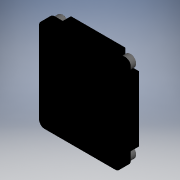
# Autodesk Inventor part: SCHUNK-Deckel ERD
Saved by Autodesk Inventor 2017.3 (Build 213256000, 256)
## iProperties
Part Number: SCHUNK-Deckel ERD
Material: Generic
Catalog Web Link: www.cadenas.de
Description: Deckel-Miniature rotary unit
Vendor: SCHUNK
Document SubType Name: Modeling
Designer: partserver
Manufacturer: SCHUNK
Mass: 53.3739 g
Surface Area: 125.943 cm^2
Volume: 53.3739 cm^3
Density: 1 g/cm^3
Appearance: PSOLRGB-0-0-0
Category: PARTsolutions
Company: SCHUNK
Title: SCHUNK-ERD
Author: Cadenas PARTsolutions
Comments: Miniature rotary unit
PSOL_IDENT_0: {$CADENAS_DATA\23d-libs\schunk\greifsysteme\drehmodule\drehmodule_elektrisch\schwenkeinheiten\miniat
PSOL_IDENT_1: ur_schwenkeinheiten\erd_dec.prj},167 {VTYP=3D},{NB=SCHUNK-Deckel ERD},{LINA=SCHUNK-ERD},{NN=Deckel},
PSOL_IDENT_2: {DATE=23.04.2020 15:23:31},{GEOMDATE=04.12.2019 08:06:04},{VERSION=},{LINEID=10},{WBVAR=},{WBNUMERIC=
PSOL_IDENT_3: }  {NB=SCHUNK-Deckel ERD},{LINA=SCHUNK-ERD},{KT=DUMMY},{TYP=ERD},{L=68.000},{B=60.000},{H1=15.000},{
PSOL_IDENT_4: H2=13.500},{AK1=40.500},{AK2=48.500},{AK3=5.000},{AK4=7.500},{AF=1.500},{SA1=58.000},{SA2=50.000},{S
PSOL_IDENT_5: D1=8.500},{SD2=4.000},{ST1=5.000},{ST2=2.500},{VBA1=20.000},{VBA2=9.500},{VBA3=5.500},{VBD1=7.000},{
PSOL_IDENT_6: VBD2=10.000},{VBT1=5.000},{VBT2=0.100},{GBA=7.500},{GBD1=2.500},{GBD2=1.500},{HALU=1.500},{LALU=24.3
PSOL_IDENT_7: 00},{BALU=9.300},{TALU=0.700}
NB: SCHUNK-Deckel ERD
NN: Deckel
NT: Miniature rotary unit
NBSYN: SCHUNK-Deckel $TYP.
LINA: SCHUNK-ERD
CATALOG: SCHUNK
TYP: ERD
L: 68
B: 60
H1: 15
H2: 13.5
AK1: 40.5
AK2: 48.5
AK3: 5
AK4: 7.5
AF: 1.5
SA1: 58
SA2: 50
SD1: 8.5
SD2: 4
ST1: 5
ST2: 2.5
VBA1: 20
VBA2: 9.5
VBA3: 5.5
VBD1: 7
VBD2: 10
VBT1: 5
VBT2: 0.1
GBA: 7.5
GBD1: 2.5
GBD2: 1.5
HALU: 1.5
LALU: 24.3
BALU: 9.3
TALU: 0.7
SUPPLIER: SCHUNK
ARTICLENO: SCHUNK-Deckel ERD
BOMINFO: SCHUNK-ERD
CREATOR: CADENAS GmbH
Autodesk Inventor part; units mm, degrees
sketch "Sketch_1" plane through (0, 0, 0) normal (0, 1, 0) x (-1, 0, 0)
  line L0 (30, -30) -> (30, 30)
  arc A0 (30, 30) -> (26, 34) centre (26, 30) ccw
  line L1 (26, 34) -> (-26, 34)
  arc A1 (-26, 34) -> (-30, 30) centre (-26, 30) ccw
  line L2 (-30, 30) -> (-30, -30)
  arc A2 (-30, -30) -> (-26, -34) centre (-26, -30) ccw
  line L3 (-26, -34) -> (26, -34)
  arc A3 (26, -34) -> (30, -30) centre (26, -30) ccw
  constraints: 8 end point, 8 point on circle, 4 centre point
extrude "Extrusion1" add sketch "Sketch_1" along normal blind 15
sketch "Sketch_2" plane through (0, 15, 0) normal (0, 1, 0) x (1, 0, 0)
  line L0 (-35, -40) -> (35, -40)
  line L1 (35, -40) -> (35, 40)
  line L2 (35, 40) -> (-35, 40)
  line L3 (-35, 40) -> (-35, -40)
  line L4 (-30, -24) -> (-25, -24)
  arc A0 (-20, -29) -> (-25, -24) centre (-25, -29) ccw
  line L5 (-20, -29) -> (-20, -34)
  line L6 (-20, -34) -> (20, -34)
  line L7 (20, -34) -> (20, -29)
  arc A1 (25, -24) -> (20, -29) centre (25, -29) ccw
  line L8 (25, -24) -> (30, -24)
  line L9 (30, -24) -> (30, 24)
  line L10 (30, 24) -> (25, 24)
  arc A2 (20, 29) -> (25, 24) centre (25, 29) ccw
  line L11 (20, 29) -> (20, 34)
  line L12 (20, 34) -> (-20, 34)
  line L13 (-20, 34) -> (-20, 29)
  arc A3 (-25, 24) -> (-20, 29) centre (-25, 29) ccw
  line L14 (-25, 24) -> (-30, 24)
  line L15 (-30, 24) -> (-30, -24)
  constraints: 32 end point, 8 point on circle, 4 centre point
extrude "Extrusion2" cut sketch "Sketch_2" against normal blind 7.5
sketch "Sketch_3" plane through (0, 0, 0) normal (1, 0, 0) x (0, 1, 0)
  line L0 (13.5, 29) -> (13.5, -34)
  line L1 (13.5, -34) -> (15, -34)
  line L2 (15, -34) -> (15, 29)
  line L3 (15, 29) -> (13.5, 29)
  constraints: 8 end point
extrude "Extrusion3" cut sketch "Sketch_3" along normal mid plane 120
sketch "Sketch_4" plane through (0, 0, 34) normal (0, 0, 1) x (1, 0, 0)
  line L0 (-20.25, 16.5) -> (-20.25, 13.5)
  line L1 (-20.25, 13.5) -> (-18.75, 15)
  line L2 (-18.75, 15) -> (18.75, 15)
  line L3 (18.75, 15) -> (20.25, 13.5)
  line L4 (20.25, 13.5) -> (20.25, 16.5)
  line L5 (20.25, 16.5) -> (-20.25, 16.5)
  constraints: 12 end point
extrude "Extrusion4" cut sketch "Sketch_4" against normal blind 5
sketch "Sketch_5" plane through (-25, 0, 0) normal (1, 0, 0) x (0, 0, -1)
  line L0 (-29, 12.5) -> (-29, 7.5)
  line L1 (-29, 7.5) -> (-33.25, 7.5)
  line L2 (-33.25, 7.5) -> (-33.25, 12)
  arc A0 (-32.75, 12.5) -> (-33.25, 12) centre (-32.75, 12) ccw
  line L3 (-32.75, 12.5) -> (-31.3, 12.5)
  line L4 (-31.3, 12.5) -> (-31, 12.2)
  line L5 (-31, 12.2) -> (-31, 10)
  line L6 (-31, 10) -> (-29, 8.7983)
  line L7 (-29, 8.7983) -> (-29, 7.5)
  constraints: 16 end point, 2 point on circle, 1 centre point
revolve "Revolution1" add sketch "Sketch_5" angle 360 about axis through (-25, 12.5, 29) along (0, 1, 0)
pattern_linear "Rectangular Pattern1" count 2 spacing 50 along (1, 0, 0) count 2 spacing 58 along (0, 0, -1) of "Revolution1"
sketch "Sketch_7" plane through (-25, 12.5, 29) normal (0, 1, 0) x (0, 0, 1)
  line L0 (-2, -1.1547) -> (0, -2.3094)
  line L1 (0, -2.3094) -> (2, -1.1547)
  line L2 (2, -1.1547) -> (2, 1.1547)
  line L3 (2, 1.1547) -> (0, 2.3094)
  line L4 (0, 2.3094) -> (-2, 1.1547)
  line L5 (-2, 1.1547) -> (-2, -1.1547)
  constraints: 12 end point
extrude "Extrusion5" cut sketch "Sketch_7" against normal blind 2.5
pattern_linear "Rectangular Pattern2" count 2 spacing 50 along (1, 0, 0) count 2 spacing 58 along (0, 0, -1) of "Extrusion5"
sketch "Sketch7" plane through (-26, 0, 34) normal (0, 0, 1) x (1, 0, 0)
  point P0 (16, 5.5)
hole "Hole1" at (-10, 5.5, 34) direction (0, 0, -1) diameter 5.9175 depth 7.3254 tip angle 118 counterbore diameter 10 counterbore depth 0.1 thread size "M7x1" class "6H" standard "ISO Metric profile"
pattern_linear "Rectangular Pattern3" count 2 spacing 20.3961 along (0.9806, 0.1961, 0) of "Hole1"
sketch "Sketch_11" plane through (0, 0, 0) normal (1, 0, 0) x (0, 1, 0)
  line L0 (7.5, 32.5494) -> (7.5, 34.1)
  line L1 (7.5, 34.1) -> (8.75, 34.1)
  line L2 (8.75, 34.1) -> (8.75, 33.8)
  line L3 (8.75, 33.8) -> (8.55, 34)
  line L4 (8.55, 34) -> (8.43, 34)
  line L5 (8.43, 34) -> (8.25, 33.82)
  line L6 (8.25, 33.82) -> (8.25, 33)
  line L7 (8.25, 33) -> (7.5, 32.5494)
  line L8 (7.5, 32.5494) -> (7.5, 34.1)
  constraints: 18 end point
revolve "Revolution2" cut sketch "Sketch_11" angle 360 about axis through (0, 7.5, 32.5494) along (0, 0, -1)
sketch "Sketch_12" plane through (0, 0, 34) normal (0, 0, 1) x (1, 0, 0)
  line L0 (-0.75, 7.067) -> (0, 6.634)
  line L1 (0, 6.634) -> (0.75, 7.067)
  line L2 (0.75, 7.067) -> (0.75, 7.933)
  line L3 (0.75, 7.933) -> (0, 8.366)
  line L4 (0, 8.366) -> (-0.75, 7.933)
  line L5 (-0.75, 7.933) -> (-0.75, 7.067)
  constraints: 12 end point
extrude "Extrusion6" cut sketch "Sketch_12" against normal blind 1
sketch "Sketch_15" plane through (30, 0, 0) normal (1, 0, 0) x (0, 0, -1)
  arc A0 (-12.15, 6.15) -> (-7.5, 1.5) centre (-7.5, 6.15) ccw
  line L0 (-7.5, 1.5) -> (7.5, 1.5)
  arc A1 (7.5, 1.5) -> (12.15, 6.15) centre (7.5, 6.15) ccw
  arc A2 (12.15, 6.15) -> (7.5, 10.8) centre (7.5, 6.15) ccw
  line L1 (7.5, 10.8) -> (-7.5, 10.8)
  arc A3 (-7.5, 10.8) -> (-12.15, 6.15) centre (-7.5, 6.15) ccw
  constraints: 8 point on circle, 4 centre point, 4 end point
extrude "Extrusion7" cut sketch "Sketch_15" against normal blind 0.7
ref_plane "geh_XY" through (0, 0, 0) normal (0, 1, 0) x (1, 0, 0)
ref_plane "geh_YZ" through (0, 0, 0) normal (1, 0, 0) x (0, 0, -1)
ref_plane "geh_ZX" through (0, 0, 0) normal (0, 0, -1) x (0, 1, 0)
ref_plane "ring_XY" through (0, 13.5, -3.5) normal (0, 1, 0) x (1, 0, 0)
ref_plane "ring_YZ" through (0, 13.5, -3.5) normal (1, 0, 0) x (0, 0, -1)
ref_plane "ring_ZX" through (0, 13.5, -3.5) normal (0, 0, -1) x (0, 1, 0)
ref_plane "typenschild_XY" through (29.3, 6.15, 0) normal (1, 0, 0) x (0, 0, -1)
ref_plane "typenschild_YZ" through (29.3, 6.15, 0) normal (0, 0, -1) x (0, 1, 0)
ref_plane "typenschild_ZX" through (29.3, 6.15, 0) normal (0, 1, 0) x (1, 0, 0)
ref_plane "vss1_XY" through (-10, 5.5, 33.9) normal (0, 0, 1) x (0, 1, 0)
ref_plane "vss1_YZ" through (-10, 5.5, 33.9) normal (0, 1, 0) x (-1, 0, 0)
ref_plane "vss1_ZX" through (-10, 5.5, 33.9) normal (-1, 0, 0) x (0, 0, 1)
ref_plane "vss2_XY" through (10, 9.5, 34) normal (0, 0, 1) x (1, 0, 0)
ref_plane "vss2_YZ" through (10, 9.5, 34) normal (1, 0, 0) x (0, 1, 0)
ref_plane "vss2_ZX" through (10, 9.5, 34) normal (0, 1, 0) x (0, 0, 1)
body "Solid1"
